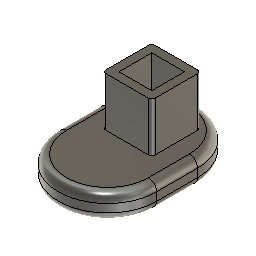
Robot Mergator (Autodesk Fusion 360 archive; units mm, degrees)
design "talpa"
Autodesk Fusion 360 part; units mm, degrees
sketch "Sketch1" plane through (0, 0, 0) normal (0, 0, 1) x (1, 0, 0)
  line L0 (30, 25) -> (30, 0)
  line L1 (-30, 25) -> (-30, 0)
  arc A0 (30, 25) -> (-30, 25) centre (0, 25) ccw
  arc A1 (-30, 0) -> (30, 0) centre (0, 0) ccw
  dimension "d1" = 60
  dimension "d2" = 60
  constraint coincident A1.centre origin
  constraint tangent L0 A1
  constraint vertical L0
  constraint tangent L1 A0
  constraint parallel L0 L1
  measures "d1" diameter of A1
  measures "d2" diameter of A0
extrude "Extrude1" add sketch "Sketch1" along normal blind 15
sketch "Sketch2" plane through (0, 0, 15) normal (0, 0, 1) x (-1, 0, 0)
  arc A0 (-30, -25) -> (30, -25) centre (0, -25) ccw
  line L0 (30, -25) -> (30, 0)
  arc A1 (30, 0) -> (-30, 0) centre (0, 0) ccw
  line L1 (-30, 0) -> (-30, -25)
  line L2 (10, -37.0225) -> (-10, -37.0225)
  line L3 (-10, -37.0225) -> (-10, -17.0225)
  line L4 (-10, -17.0225) -> (10, -17.0225)
  line L5 (10, -17.0225) -> (10, -37.0225)
  line L6 (15, -42.0225) -> (-15, -42.0225)
  line L7 (-15, -42.0225) -> (-15, -12.0225)
  line L8 (-15, -12.0225) -> (15, -12.0225)
  line L9 (15, -12.0225) -> (15, -42.0225)
  constraint horizontal L2
  constraint vertical L3
  constraint horizontal L4
  constraint vertical L5
  constraint horizontal L6
  constraint vertical L7
  constraint horizontal L8
  constraint vertical L9
fillet "Fillet1" radius 5 8 edges at (0, 55, 15) (-30, 12.5, 15) (0, -30, 15) (30, 12.5, 15) (30, 12.5, 0) (0, 55, 0) (-30, 12.5, 0) (0, -30, 0)
extrude "Extrude3" add sketch "Sketch2" along normal blind 30 contours L6 L7 L8 L9
fillet "Fillet2" radius 2 4 edges at (15, 12.0225, 30) (-15, 12.0225, 30) (-15, 42.0225, 30) (15, 42.0225, 30)
